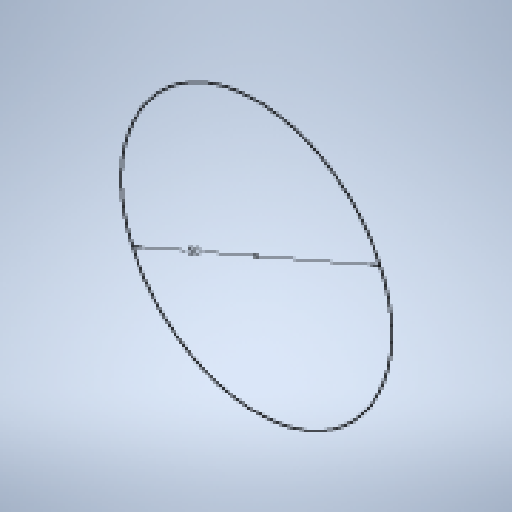
# Autodesk Inventor part: Part1
Saved by Autodesk Inventor 2024.2 (Build 282272000, 272)
## iProperties
Created: 2024-04-10
Part Number: Part1
Material: Generic
Document SubType Name: Sheet Metal
Designer: admin
Density: 1 g/cm^3
Sheet Metal Rule: Default
Appearance: Default
Author: admin
Autodesk Inventor part; units mm, degrees
ref_plane "YZ Plane" through (0, 0, 0) normal (1, 0, 0) x (0, 1, 0)
ref_plane "XZ Plane" through (0, 0, 0) normal (0, 1, 0) x (-1, 0, 0)
ref_plane "XY Plane" through (0, 0, 0) normal (0, 0, 1) x (1, 0, 0)
sketch "Sketch1" plane through (0, 0, 0) normal (0, 0, 1) x (1, 0, 0)
  circle A0 centre (0, 0) radius 25
  line L0 (-25, 0) -> (-35, 0)
  line L1 (25, 0) -> (35, 0)
  line L2 (-35, 0) -> (-46, -50)
  line L3 (-46, -50) -> (-46, -60)
  line L4 (-46, -60) -> (46, -60)
  line L5 (46, -60) -> (46, -50)
  line L6 (46, -50) -> (35, 0)
  point P0 (30, 0)
  point P1 (-30, 0)
  point P2 (0, -60)
  dimension "d0" = 50
  dimension "d1" = 10
  dimension "d2" = 10
  dimension "d3" = 60
  dimension "d4" = 92
  constraints: 14 end point, 4 perpendicular, 3 midpoint, 2 horizontal, 2 horizontal alignment, 2 point on circle, 1 centre point, 1 coincident, 1 vertical, 1 vertical alignment
  measures "d0" diameter of A0
  measures "d1" distance of L0.start L0.end
  measures "d2" distance of L1.start L1.end
  measures "d3" distance from line of L4 point (0, 0)
  measures "d4" distance of L3.end L4.end
extrude "Extrusion1" add sketch "Sketch1" along normal blind 3 contours L1 L6 L5 L4 L3 L2 L0 A0
equation "\"BendRadius\" = Thickness"
equation "\"BendReliefWidth\" = Thickness"
equation "\"BendReliefDepth\" = 0.5 * Thickness"
equation "\"CornerReliefSize\" = 4 * Thickness"
equation "\"MinimumRemnant\" = 2 * Thickness"
equation "\"TransitionRadius\" = BendRadius"
equation "\"JacobiRadiusSize\" = BendRadius"
equation "\"GapSize\" = Thickness"
equation "\"Thickness\" = 3"
body "Solid1"
